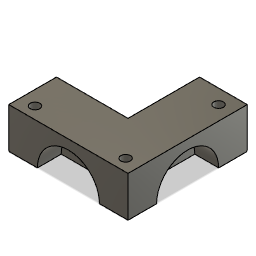
Lock2 (Autodesk Fusion 360 design; units mm, degrees)
Autodesk Fusion 360 part; units mm, degrees
note: some values were not read from the file. Set by a fixed rule: which sketch regions a step uses.
sketch "Sketch1" plane through (0, 0, 0) normal (0, 1, 0) x (1, 0, 0)
  line L0 (0, 0) -> (25, 0)
  line L1 (25, 0) -> (25, 25)
  line L2 (25, 25) -> (15, 25)
  line L3 (0, 10) -> (0, 0)
  line L4 (15, 25) -> (15, 10)
  line L5 (15, 10) -> (0, 10)
  dimension "d13" = 25
  dimension "d14" = 25
  dimension "d15" = 15
  constraint horizontal L0
  constraint vertical L1
  constraint horizontal L2
  constraint vertical L3
  constraint coincident L0.start L3.end
  constraint vertical L4
  constraint horizontal L5
  measures "d13" distance of L0 L2
  measures "d14" distance of L1 L3
  measures "d15" distance of L2.end L4.end
extrude "Extrude1" add sketch "Sketch1" along normal blind 8.5
sketch "Sketch2" plane through (25, 0, 0) normal (1, 0, 0) x (0, 0, -1)
  line L0 (0, 0) -> (25, 0)
  line L1 (25, 0) -> (25, 8.5)
  line L2 (25, 8.5) -> (0, 8.5)
  line L3 (0, 8.5) -> (0, 0)
  arc A0 (19, 0) -> (6, 0) centre (12.5, 0) ccw
  line L4 (6, 0) -> (19, 0)
  dimension "d5" = 13
  constraint midpoint L0 A0.centre
  constraint coincident L0 A0.end
  constraint coincident L0 A0.start
  measures "d5" diameter of A0
extrude "Extrude2" cut sketch "Sketch2" against normal blind 5 contours L0 A0 L4
sketch "Sketch3" plane through (0, 0, 0) normal (0, 0, 1) x (1, 0, 0)
  line L0 (0, 0) -> (25, 0)
  line L1 (25, 0) -> (25, 8.5)
  line L2 (25, 8.5) -> (0, 8.5)
  line L3 (0, 8.5) -> (0, 0)
  arc A0 (19, 0) -> (6, 0) centre (12.5, 0) ccw
  line L4 (6, 0) -> (19, 0)
  dimension "d8" = 13
  constraint midpoint L0 A0.centre
  constraint coincident L0 A0.end
  constraint coincident L0 A0.start
  measures "d8" diameter of A0
extrude "Extrude3" cut sketch "Sketch3" against normal blind 5 contours L0 A0 L4
sketch "Sketch4" plane through (0, 0, 0) normal (0, -1, 0) x (1, 0, 0)
  line L0 (19, 0) -> (19, -5)
  line L1 (19, -5) -> (6, -5)
  line L2 (6, -5) -> (6, 0)
  line L3 (6, 0) -> (0, 0)
  line L4 (0, 0) -> (0, -10)
  line L5 (0, -10) -> (15, -10)
  line L6 (15, -10) -> (15, -25)
  line L7 (15, -25) -> (25, -25)
  line L8 (25, -25) -> (25, -19)
  line L9 (25, -19) -> (20, -19)
  line L10 (20, -19) -> (20, -6)
  line L11 (20, -6) -> (25, -6)
  line L12 (25, -6) -> (25, 0)
  line L13 (25, 0) -> (19, 0)
  circle A0 centre (3, -2.5) radius 1
  line L14 (0, -2.5) -> (25, -2.5) construction
  line L15 (22, 0) -> (22, -25) construction
  line L16 (25, -22) -> (24.6457, -22)
  line L17 (24.6457, -22) -> (15, -22) construction
  line L18 (3, 0) -> (3, -10) construction
  circle A1 centre (22, -22) radius 1
  circle A2 centre (22, -2.5) radius 1
  dimension "d16" = 2
  constraint coincident L12 L14.end
  constraint perpendicular L12 L14
  constraint midpoint L13 L15.start
  constraint coincident L7 L15.end
  constraint perpendicular L7 L15
  constraint midpoint L8 L16.start
  constraint perpendicular L8 L16
  constraint coincident L6 L17.end
  constraint perpendicular L6 L17
  constraint coincident L4 L14.start
  constraint midpoint L3 L18.start
  constraint coincident L5 L18.end
  constraint perpendicular L5 L18
  constraint coincident A0.centre L18
  constraint coincident A0.centre L14
  constraint coincident L15 A1.centre
  constraint coincident L17 A1.centre
  constraint equal A0 A1
  constraint coincident L14 A2.centre
  constraint coincident L15 A2.centre
  constraint equal A0 A2
  measures "d16" diameter of A0
extrude "Extrude4" cut sketch "Sketch4" against normal through all contours A0 | A1 | A2
fillet "Fillet1" radius 0.2 2 edges at (0, 0, -5) (20, 0, -25)
